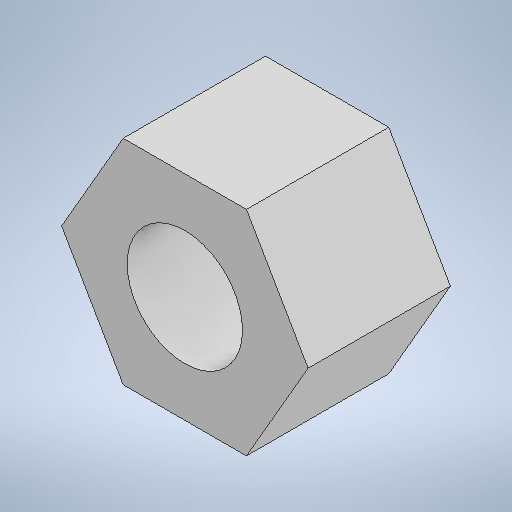
# Autodesk Inventor part: Tool-Lock-Knob
Saved by Autodesk Inventor 2025.3 (Build 293356030, 356C)
## iProperties
Created: 2025-10-10
Part Number: Tool-Lock-Knob
Material: Generic
Document SubType Name: Modeling
Designer: tvoko
Density: 1 g/cm^3
Appearance: Default
Author: tvoko
Autodesk Inventor part; units mm, degrees
ref_plane "YZ Plane" through (0, 0, 0) normal (1, 0, 0) x (0, 1, 0)
ref_plane "XZ Plane" through (0, 0, 0) normal (0, 1, 0) x (-1, 0, 0)
ref_plane "XY Plane" through (0, 0, 0) normal (0, 0, 1) x (1, 0, 0)
sketch "Sketch1" plane through (0, 0, 0) normal (0, 0, 1) x (1, 0, 0)
  circle A0 centre (0, 0) radius 4.05
  line L0 (-4.3301, -7.5) -> (-8.6603, 0)
  line L1 (-8.6603, 0) -> (-4.3301, 7.5)
  line L2 (-4.3301, 7.5) -> (4.3301, 7.5)
  line L3 (4.3301, 7.5) -> (8.6603, 0)
  line L4 (8.6603, 0) -> (4.3301, -7.5)
  line L5 (4.3301, -7.5) -> (-4.3301, -7.5)
  dimension "d0" = 8.1
  dimension "d1" = 15
  constraints: 12 end point, 2 coincident, 1 centre point, 1 horizontal, 13 other
  measures "d0" diameter of A0
  measures "d1" distance between parallel lines of L5 L2
extrude "Extrusion1" add sketch "Sketch1" along normal blind 10
body "Solid1"
